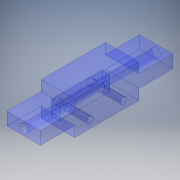
# Autodesk Inventor part: SliderSlide2r
Saved by Autodesk Inventor 2019 (Build 230136000, 136)
## iProperties
Created: 2019-10-06
Part Number: SliderSlide2r
Material: Generic
Document SubType Name: Modeling
Designer: james
Density: 1 g/cm^3
Appearance: Clear - Blue
Author: james
Autodesk Inventor part; units mm, degrees
ref_plane "YZ Plane" through (0, 0, 0) normal (1, 0, 0) x (0, 1, 0)
ref_plane "XZ Plane" through (0, 0, 0) normal (0, 1, 0) x (-1, 0, 0)
ref_plane "XY Plane" through (0, 0, 0) normal (0, 0, 1) x (1, 0, 0)
sketch "Sketch1" plane through (0, 0, 0) normal (0, 0, 1) x (1, 0, 0)
  line L0 (-42.4234, 22.9681) -> (-17.0234, 22.9681)
  line L1 (-17.0234, 22.9681) -> (-17.0234, -2.4319)
  line L2 (-17.0234, -2.4319) -> (-42.4234, -2.4319)
  line L3 (-42.4234, -2.4319) -> (-42.4234, 22.9681)
  point P0 (0, 0)
  dimension "d0" = 25.4
  dimension "d1" = 25.4
  constraints: 8 end point, 2 parallel, 1 horizontal, 1 perpendicular
  measures "d0" distance of L1.end L2.end
  measures "d1" distance of L0.end L1.end
extrude "Extrusion1" add sketch "Sketch1" along normal blind 48.768
sketch "Sketch2" plane through (-17.0234, -2.4319, 0) normal (1, 0, 0) x (0, 0, -1)
  line L0 (-48.768, 17.526) -> (-48.768, 7.874)
  line L1 (-48.768, 7.874) -> (-74.676, 7.874)
  line L2 (-74.676, 7.874) -> (-74.676, 17.526)
  line L3 (-74.676, 17.526) -> (-48.768, 17.526)
  line L4 (-48.768, 0) -> (-48.768, 25.4) projected
  line L5 (0, 0) -> (-48.768, 0) projected
  line L6 (0, 25.4) -> (-48.768, 25.4) projected
  point P0 (0, 2.4319)
  dimension "d4" = 25.908
  dimension "d94" = 7.874
  dimension "d95" = 7.874
  constraints: 8 end point, 3 perpendicular, 2 point on line, 1 vertical
  measures "d4" distance between parallel lines of L0 L2
  measures "d94" distance between parallel lines of L5 L1
  measures "d95" distance between parallel lines of L3 L6
extrude "Extrusion2" add sketch "Sketch2" against normal blind 25.4
sketch "Sketch3" plane through (-17.0234, -2.4319, 0) normal (1, 0, 0) x (0, 0, -1)
  line L0 (0, 17.526) -> (0, 7.874)
  line L1 (0, 7.874) -> (25.908, 7.874)
  line L2 (25.908, 7.874) -> (25.908, 17.526)
  line L3 (25.908, 17.526) -> (0, 17.526)
  line L4 (-74.676, 7.874) -> (-48.768, 7.874) projected
  line L5 (-48.768, 17.526) -> (-74.676, 17.526) projected
  line L6 (0, 25.4) -> (0, 0) projected
  line L7 (0, 0) -> (-48.768, 0) projected
  line L8 (0, 25.4) -> (-48.768, 25.4) projected
  point P0 (0, 2.4319)
  point P1 (0, 22.86)
  point P2 (-55.88, 7.62)
  point P3 (-55.88, 17.78)
  point P4 (-48.768, 7.874)
  dimension "d20" = 9.652
  dimension "d23" = 9.652
  dimension "d92" = 7.874
  dimension "d96" = 25.908
  dimension "d97" = 7.874
  constraints: 8 end point, 3 perpendicular, 3 point on line, 1 vertical, 2 other
  measures "d23" distance of L1.end L2.end
  measures "d92" distance between parallel lines of L7 L1
  measures "d96" distance between parallel lines of L2 L0
  measures "d97" distance between parallel lines of L3 L8
extrude "Extrusion3" add sketch "Sketch3" against normal blind 25.4
sketch "Sketch4" plane through (-17.0234, 5.4421, 74.676) normal (0, 0, 1) x (1, 0, 0)
  line L0 (0, 9.652) -> (-25.4, 9.652) projected
  line L1 (-25.4, 0) -> (-25.4, 9.652) projected
  point P0 (17.0234, -5.4421)
  point P1 (-12.7, 4.572)
  dimension "d26" = 5.08
  dimension "d27" = 12.7
  measures "d26" distance from line of point (-12.7, 4.572) L0
  measures "d27" distance from line of L1 point (-12.7, 4.572)
hole "Hole1" at (-29.7234, 10.0141, 74.676) direction (0, 0, -1) diameter 6.477 end through all
sketch "Sketch5" plane through (-17.0234, 22.9681, 48.768) normal (1, 0, 0) x (0, 0, -1)
  line L0 (48.768, -25.4) -> (0, -25.4) projected
  point P0 (48.768, -22.9681)
  point P1 (11.684, -19.812)
  point P2 (37.084, -19.812)
  dimension "d35" = 5.588
  dimension "d36" = 5.588
  dimension "d37" = 11.684
  dimension "d38" = 11.684
  dimension "d93" = 25.4
  measures "d35" distance from line of L0 point (37.084, -19.812)
  measures "d36" distance from line of L0 point (11.684, -19.812)
  measures "d37" horizontal distance of L0.end point (11.684, -19.812)
  measures "d38" horizontal distance of L0.start point (37.084, -19.812)
  measures "d93" distance of point (37.084, -19.812) point (11.684, -19.812)
hole "Hole2" at (-17.0234, 3.1561, 37.084) at (-17.0234, 3.1561, 11.684) direction (-1, 0, 0) diameter 4.9784 end through all thread size "1/4-20 UNC" class "2B" standard "ANSI Unified Screw Threads"
sketch "Sketch19" plane through (-42.4234, -2.4319, 0) normal (0, -1, 0) x (1, 0, 0)
  line L0 (8.54, 43.688) -> (2.54, 43.688)
  line L1 (2.54, 43.688) -> (2.54, 5.08)
  line L2 (2.54, 5.08) -> (8.54, 5.08)
  line L3 (8.54, 5.08) -> (8.54, 43.688)
  line L4 (25.4, 0) -> (0, 0) projected
  line L5 (0, 48.768) -> (25.4, 48.768) projected
  line L6 (0, 0) -> (0, 48.768) projected
  point P0 (42.4234, 0)
  dimension "d98" = 6
  dimension "d99" = 5.08
  dimension "d100" = 5.08
  dimension "d101" = 2.54
  constraints: 8 end point, 2 parallel, 1 horizontal, 1 perpendicular
  measures "d98" distance between parallel lines of L1 L3
  measures "d99" distance between parallel lines of L4 L2
  measures "d100" distance between parallel lines of L5 L0
  measures "d101" distance between parallel lines of L6 L1
extrude "Extrusion13" cut sketch "Sketch19" against normal blind 11.213
body "Solid1"
